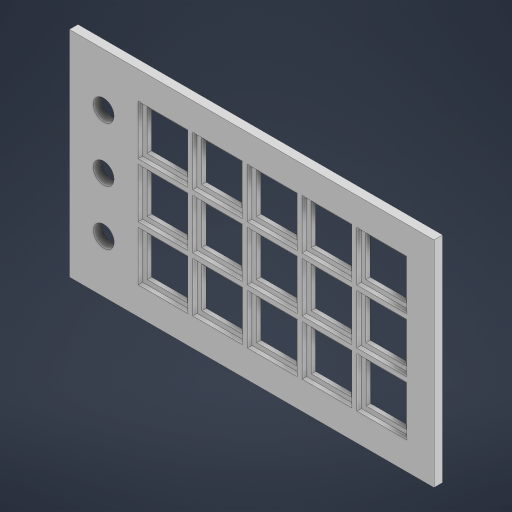
# Autodesk Inventor part: keypadTop
Saved by Autodesk Inventor 2024.3 (Build 283343000, 343)
## iProperties
Created: 2025-12-23
Part Number: keypadTop
Material: Generic
Document SubType Name: Modeling
Designer: zokur
Density: 1 g/cm^3
Appearance: Default
Author: zokur
Autodesk Inventor part; units mm, degrees
ref_plane "YZ Plane" through (0, 0, 0) normal (1, 0, 0) x (0, 1, 0)
ref_plane "XZ Plane" through (0, 0, 0) normal (0, 1, 0) x (-1, 0, 0)
ref_plane "XY Plane" through (0, 0, 0) normal (0, 0, 1) x (1, 0, 0)
sketch "Sketch1" plane through (0, 0, 0) normal (0, 0, 1) x (1, 0, 0)
  line L0 (0, 0) -> (126.85, 0)
  line L1 (126.85, 0) -> (126.85, 74.6)
  line L2 (126.85, 74.6) -> (0, 74.6)
  line L3 (0, 74.6) -> (0, 0)
  line L4 (100, 64.95) -> (117.3, 64.95)
  line L5 (117.3, 64.95) -> (117.3, 47.65)
  line L6 (117.3, 47.65) -> (100, 47.65)
  line L7 (100, 47.65) -> (100, 64.95)
  line L8 (100, 45.95) -> (117.3, 45.95)
  line L9 (117.3, 45.95) -> (117.3, 28.65)
  line L10 (117.3, 28.65) -> (100, 28.65)
  line L11 (100, 28.65) -> (100, 45.95)
  line L12 (100.05, 26.95) -> (117.35, 26.95)
  line L13 (117.35, 26.95) -> (117.35, 9.65)
  line L14 (117.35, 9.65) -> (100.05, 9.65)
  line L15 (100.05, 9.65) -> (100.05, 26.95)
  line L16 (80.95, 65.0676) -> (98.25, 65.0676)
  line L17 (98.25, 65.0676) -> (98.25, 47.7676)
  line L18 (98.25, 47.7676) -> (80.95, 47.7676)
  line L19 (80.95, 47.7676) -> (80.95, 65.0676)
  line L20 (80.95, 46.0676) -> (98.25, 46.0676)
  line L21 (98.25, 46.0676) -> (98.25, 28.7676)
  line L22 (98.25, 28.7676) -> (80.95, 28.7676)
  line L23 (80.95, 28.7676) -> (80.95, 46.0676)
  line L24 (98.3, 27.0676) -> (98.3, 9.7676)
  line L25 (81, 27.0676) -> (98.3, 27.0676)
  line L26 (81, 9.7676) -> (81, 27.0676)
  line L27 (98.3, 9.7676) -> (81, 9.7676)
  line L28 (61.95, 64.95) -> (79.25, 64.95)
  line L29 (79.25, 64.95) -> (79.25, 47.65)
  line L30 (79.25, 47.65) -> (61.95, 47.65)
  line L31 (61.95, 47.65) -> (61.95, 64.95)
  line L32 (61.95, 45.95) -> (79.25, 45.95)
  line L33 (79.25, 45.95) -> (79.25, 28.65)
  line L34 (79.25, 28.65) -> (61.95, 28.65)
  line L35 (61.95, 28.65) -> (61.95, 45.95)
  line L36 (79.3, 26.95) -> (79.3, 9.65)
  line L37 (62, 26.95) -> (79.3, 26.95)
  line L38 (62, 9.65) -> (62, 26.95)
  line L39 (79.3, 9.65) -> (62, 9.65)
  line L40 (60.2, 28.7676) -> (42.9, 28.7676)
  line L41 (42.9, 28.7676) -> (42.9, 46.0676)
  line L42 (60.2, 46.0676) -> (60.2, 28.7676)
  line L43 (42.9, 46.0676) -> (60.2, 46.0676)
  line L44 (60.2, 47.7676) -> (42.9, 47.7676)
  line L45 (60.2, 65.0676) -> (60.2, 47.7676)
  line L46 (42.9, 47.7676) -> (42.9, 65.0676)
  line L47 (42.9, 65.0676) -> (60.2, 65.0676)
  line L48 (42.95, 27.0676) -> (60.25, 27.0676)
  line L49 (42.95, 9.7676) -> (42.95, 27.0676)
  line L50 (60.25, 9.7676) -> (42.95, 9.7676)
  line L51 (60.25, 27.0676) -> (60.25, 9.7676)
  line L52 (41.2, 64.95) -> (41.2, 47.65)
  line L53 (23.9, 64.95) -> (41.2, 64.95)
  line L54 (23.9, 47.65) -> (23.9, 64.95)
  line L55 (41.2, 47.65) -> (23.9, 47.65)
  line L56 (23.9, 45.95) -> (41.2, 45.95)
  line L57 (41.2, 45.95) -> (41.2, 28.65)
  line L58 (23.9, 28.65) -> (23.9, 45.95)
  line L59 (41.2, 28.65) -> (23.9, 28.65)
  line L60 (23.95, 26.95) -> (41.25, 26.95)
  line L61 (41.25, 9.65) -> (23.95, 9.65)
  line L62 (41.25, 26.95) -> (41.25, 9.65)
  line L63 (23.95, 9.65) -> (23.95, 26.95)
  circle A0 centre (11.95, 56.3) radius 3.6
  circle A1 centre (11.95, 37.3) radius 3.6
  circle A2 centre (12, 18.3) radius 3.6
  point P0 (108.65, 45.95)
  point P1 (108.7, 26.95)
  point P2 (89.6, 46.0676)
  point P3 (89.65, 27.0676)
  point P4 (70.6, 45.95)
  point P5 (70.65, 26.95)
  point P6 (51.55, 46.0676)
  point P7 (51.6, 27.0676)
  point P8 (32.55, 45.95)
  point P9 (32.6, 26.95)
  dimension "d0" = 74.6
  dimension "d1" = 126.85
  dimension "d2" = 17.3
  dimension "d3" = 17.3
  dimension "d4" = 9.55
  dimension "d5" = 9.65
  dimension "d6" = 17.3
  dimension "d7" = 17.3
  dimension "d8" = 9.55
  dimension "d9" = 1.7
  dimension "d10" = 17.3
  dimension "d11" = 17.3
  dimension "d12" = 1.7
  dimension "d13" = 9.5
  dimension "d14" = 17.3
  dimension "d15" = 17.3
  dimension "d16" = 17.3
  dimension "d17" = 17.3
  dimension "d18" = 1.7
  dimension "d19" = 17.3
  dimension "d20" = 17.3
  dimension "d21" = 1.7
  dimension "d22" = 1.7
  dimension "d23" = 28.6
  dimension "d24" = 28.6
  dimension "d25" = 0.1176
  dimension "d26" = 17.3
  dimension "d27" = 17.3
  dimension "d28" = 17.3
  dimension "d29" = 17.3
  dimension "d30" = 1.7
  dimension "d31" = 17.3
  dimension "d32" = 17.3
  dimension "d33" = 1.7
  dimension "d34" = 17.3
  dimension "d35" = 17.3
  dimension "d36" = 17.3
  dimension "d37" = 17.3
  dimension "d38" = 1.7
  dimension "d39" = 17.3
  dimension "d40" = 17.3
  dimension "d41" = 1.7
  dimension "d42" = 1.7
  dimension "d43" = 0.1176
  dimension "d44" = 1.7
  dimension "d45" = 1.7
  dimension "d46" = 9.65
  dimension "d47" = 47.6
  dimension "d48" = 66.65
  dimension "d49" = 66.65
  dimension "d50" = 17.3
  dimension "d51" = 17.3
  dimension "d52" = 17.3
  dimension "d53" = 17.3
  dimension "d54" = 1.7
  dimension "d55" = 17.3
  dimension "d56" = 17.3
  dimension "d57" = 1.7
  dimension "d58" = 1.7
  dimension "d59" = 9.65
  dimension "d60" = 85.65
  dimension "d61" = 85.65
  dimension "d62" = 7.2
  dimension "d63" = 11.95
  constraints: 128 end point, 32 parallel, 16 horizontal, 16 perpendicular, 10 midpoint, 3 centre point
  measures "d0" distance of L0.end L1.end
  measures "d1" distance of L1.end L2.end
  measures "d2" distance of L5.end L6.end
  measures "d3" distance of L6.end L4.start
  measures "d4" distance between parallel lines of L1 L5
  measures "d5" distance between parallel lines of L2 L4
  measures "d6" distance of L9.end L10.end
  measures "d7" distance of L10.end L8.start
  measures "d8" distance between parallel lines of L1 L9
  measures "d9" distance from line of point (108.65, 45.95) L6
  measures "d10" distance of L13.end L15.start
  measures "d11" distance of L15.start L12.start
  measures "d12" distance between parallel lines of L12 L10
  measures "d13" distance between parallel lines of L1 L13
  measures "d14" distance of L18.start L18.end
  measures "d15" distance of L18.end L19.end
  measures "d16" distance of L22.start L22.end
  measures "d17" distance of L22.end L23.end
  measures "d18" distance from line of point (89.6, 46.068) L18
  measures "d19" distance of L27.start L26.start
  measures "d20" distance of L26.start L25.start
  measures "d21" distance between parallel lines of L25 L22
  measures "d22" distance between parallel lines of L11 L24
  measures "d23" distance between parallel lines of L17 L1
  measures "d24" distance between parallel lines of L21 L1
  measures "d25" distance between parallel lines of L27 L14
  measures "d26" distance of L30.start L30.end
  measures "d27" distance of L30.end L28.start
  measures "d28" distance of L33.end L35.start
  measures "d29" distance of L35.start L32.start
  measures "d30" distance from line of point (70.6, 45.95) L30
  measures "d31" distance of L36.end L38.start
  measures "d32" distance of L38.start L37.start
  measures "d33" distance between parallel lines of L37 L34
  measures "d34" distance of L45.end L46.start
  measures "d35" distance of L46.start L47.start
  measures "d36" distance of L42.end L41.start
  measures "d37" distance of L41.start L43.start
  measures "d38" distance from line of point (51.55, 46.068) L44
  measures "d39" distance of L50.start L50.end
  measures "d40" distance of L50.end L48.start
  measures "d41" distance between parallel lines of L48 L40
  measures "d42" distance between parallel lines of L35 L51
  measures "d43" distance between parallel lines of L50 L39
  measures "d44" distance between parallel lines of L26 L36
  measures "d45" distance between parallel lines of L23 L33
  measures "d46" distance between parallel lines of L2 L28
  measures "d47" distance between parallel lines of L29 L1
  measures "d48" distance between parallel lines of L45 L1
  measures "d49" distance between parallel lines of L42 L1
  measures "d50" distance of L55.start L55.end
  measures "d51" distance of L55.end L53.start
  measures "d52" distance of L57.end L59.end
  measures "d53" distance of L59.end L56.start
  measures "d54" distance from line of point (32.55, 45.95) L55
  measures "d55" distance of L62.end L61.end
  measures "d56" distance of L61.end L60.start
  measures "d57" distance between parallel lines of L60 L59
  measures "d58" distance between parallel lines of L49 L62
  measures "d59" distance between parallel lines of L0 L61
  measures "d60" distance between parallel lines of L52 L1
  measures "d61" distance between parallel lines of L57 L1
  measures "d62" diameter of A0
  measures "d63" distance from line of L54 A0.centre
extrude "Extrusion1" add sketch "Sketch1" along normal blind 3
sketch "Sketch3" plane through (0, 0, 0) normal (0, 0, -1) x (-1, 0, 0)
  line L0 (-126.85, 0) -> (-126.85, 74.6) projected
  line L1 (0, 0) -> (-126.85, 0) projected
  line L2 (0, 74.6) -> (0, 0) projected
  line L3 (-126.85, 74.6) -> (0, 74.6) projected
  circle A0 centre (-11.95, 56.3) radius 3.6 projected
  circle A1 centre (-11.95, 37.3) radius 3.6 projected
  circle A2 centre (-12, 18.3) radius 3.6 projected
  line L4 (-41.25, 26.95) -> (-41.25, 9.65) projected
  line L5 (-23.95, 26.95) -> (-41.25, 26.95) projected
  line L6 (-23.95, 9.65) -> (-23.95, 26.95) projected
  line L7 (-41.25, 9.65) -> (-23.95, 9.65) projected
  line L8 (-41.2, 47.65) -> (-23.9, 47.65) projected
  line L9 (-41.2, 64.95) -> (-41.2, 47.65) projected
  line L10 (-23.9, 64.95) -> (-41.2, 64.95) projected
  line L11 (-23.9, 47.65) -> (-23.9, 64.95) projected
  line L12 (-41.2, 45.95) -> (-41.2, 28.65) projected
  line L13 (-23.9, 45.95) -> (-41.2, 45.95) projected
  line L14 (-23.9, 28.65) -> (-23.9, 45.95) projected
  line L15 (-41.2, 28.65) -> (-23.9, 28.65) projected
  line L16 (-62, 26.95) -> (-79.3, 26.95) projected
  line L17 (-62, 9.65) -> (-62, 26.95) projected
  line L18 (-79.3, 9.65) -> (-62, 9.65) projected
  line L19 (-79.3, 26.95) -> (-79.3, 9.65) projected
  line L20 (-42.95, 27.0676) -> (-60.25, 27.0676) projected
  line L21 (-42.95, 9.7676) -> (-42.95, 27.0676) projected
  line L22 (-60.25, 9.7676) -> (-42.95, 9.7676) projected
  line L23 (-60.25, 27.0676) -> (-60.25, 9.7676) projected
  line L24 (-61.95, 45.95) -> (-79.25, 45.95) projected
  line L25 (-61.95, 28.65) -> (-61.95, 45.95) projected
  line L26 (-79.25, 28.65) -> (-61.95, 28.65) projected
  line L27 (-79.25, 45.95) -> (-79.25, 28.65) projected
  line L28 (-79.25, 47.65) -> (-61.95, 47.65) projected
  line L29 (-79.25, 64.95) -> (-79.25, 47.65) projected
  line L30 (-61.95, 64.95) -> (-79.25, 64.95) projected
  line L31 (-61.95, 47.65) -> (-61.95, 64.95) projected
  line L32 (-42.9, 46.0676) -> (-60.2, 46.0676) projected
  line L33 (-42.9, 28.7676) -> (-42.9, 46.0676) projected
  line L34 (-60.2, 28.7676) -> (-42.9, 28.7676) projected
  line L35 (-60.2, 46.0676) -> (-60.2, 28.7676) projected
  line L36 (-60.2, 65.0676) -> (-60.2, 47.7676) projected
  line L37 (-42.9, 65.0676) -> (-60.2, 65.0676) projected
  line L38 (-42.9, 47.7676) -> (-42.9, 65.0676) projected
  line L39 (-60.2, 47.7676) -> (-42.9, 47.7676) projected
  line L40 (-81, 27.0676) -> (-98.3, 27.0676) projected
  line L41 (-81, 9.7676) -> (-81, 27.0676) projected
  line L42 (-98.3, 9.7676) -> (-81, 9.7676) projected
  line L43 (-98.3, 27.0676) -> (-98.3, 9.7676) projected
  line L44 (-98.25, 47.7676) -> (-80.95, 47.7676) projected
  line L45 (-98.25, 65.0676) -> (-98.25, 47.7676) projected
  line L46 (-80.95, 65.0676) -> (-98.25, 65.0676) projected
  line L47 (-80.95, 47.7676) -> (-80.95, 65.0676) projected
  line L48 (-98.25, 28.7676) -> (-80.95, 28.7676) projected
  line L49 (-98.25, 46.0676) -> (-98.25, 28.7676) projected
  line L50 (-80.95, 46.0676) -> (-98.25, 46.0676) projected
  line L51 (-80.95, 28.7676) -> (-80.95, 46.0676) projected
  line L52 (-117.35, 26.95) -> (-117.35, 9.65) projected
  line L53 (-100.05, 26.95) -> (-117.35, 26.95) projected
  line L54 (-100.05, 9.65) -> (-100.05, 26.95) projected
  line L55 (-117.35, 9.65) -> (-100.05, 9.65) projected
  line L56 (-100, 45.95) -> (-117.3, 45.95) projected
  line L57 (-100, 28.65) -> (-100, 45.95) projected
  line L58 (-117.3, 28.65) -> (-100, 28.65) projected
  line L59 (-117.3, 45.95) -> (-117.3, 28.65) projected
  line L60 (-100, 64.95) -> (-117.3, 64.95) projected
  line L61 (-100, 47.65) -> (-100, 64.95) projected
  line L62 (-117.3, 47.65) -> (-100, 47.65) projected
  line L63 (-117.3, 64.95) -> (-117.3, 47.65) projected
  line L64 (-115.65, 63.3) -> (-115.65, 49.3) projected
  line L65 (-101.65, 63.3) -> (-115.65, 63.3) projected
  line L66 (-101.65, 49.3) -> (-101.65, 63.3) projected
  line L67 (-115.65, 49.3) -> (-101.65, 49.3) projected
  line L68 (-96.6, 63.4176) -> (-96.6, 49.4176) projected
  line L69 (-82.6, 63.4176) -> (-96.6, 63.4176) projected
  line L70 (-82.6, 49.4176) -> (-82.6, 63.4176) projected
  line L71 (-96.6, 49.4176) -> (-82.6, 49.4176) projected
  line L72 (-77.6, 63.3) -> (-77.6, 49.3) projected
  line L73 (-63.6, 63.3) -> (-77.6, 63.3) projected
  line L74 (-63.6, 49.3) -> (-63.6, 63.3) projected
  line L75 (-77.6, 49.3) -> (-63.6, 49.3) projected
  line L76 (-58.55, 63.4176) -> (-58.55, 49.4176) projected
  line L77 (-44.55, 63.4176) -> (-58.55, 63.4176) projected
  line L78 (-44.55, 49.4176) -> (-44.55, 63.4176) projected
  line L79 (-58.55, 49.4176) -> (-44.55, 49.4176) projected
  line L80 (-39.55, 63.3) -> (-39.55, 49.3) projected
  line L81 (-25.55, 63.3) -> (-39.55, 63.3) projected
  line L82 (-25.55, 49.3) -> (-25.55, 63.3) projected
  line L83 (-39.55, 49.3) -> (-25.55, 49.3) projected
  line L84 (-25.55, 44.3) -> (-39.55, 44.3) projected
  line L85 (-39.55, 44.3) -> (-39.55, 30.3) projected
  line L86 (-39.55, 30.3) -> (-25.55, 30.3) projected
  line L87 (-23.9, 28.65) -> (-23.9, 45.95) projected
  line L88 (-25.55, 30.3) -> (-25.55, 44.3) projected
  line L89 (-58.55, 30.4176) -> (-44.55, 30.4176) projected
  line L90 (-58.55, 44.4176) -> (-58.55, 30.4176) projected
  line L91 (-44.55, 44.4176) -> (-58.55, 44.4176) projected
  line L92 (-44.55, 30.4176) -> (-44.55, 44.4176) projected
  line L93 (-42.9, 28.7676) -> (-42.9, 46.0676) projected
  line L94 (-44.6, 25.4176) -> (-58.6, 25.4176) projected
  line L95 (-58.6, 25.4176) -> (-58.6, 11.4176) projected
  line L96 (-58.6, 11.4176) -> (-44.6, 11.4176) projected
  line L97 (-44.6, 11.4176) -> (-44.6, 25.4176) projected
  line L98 (-39.6, 25.3) -> (-39.6, 11.3) projected
  line L99 (-25.6, 25.3) -> (-39.6, 25.3) projected
  line L100 (-39.6, 11.3) -> (-25.6, 11.3) projected
  line L101 (-25.6, 11.3) -> (-25.6, 25.3) projected
  line L102 (-23.95, 9.65) -> (-23.95, 26.95) projected
  line L103 (-23.95, 26.95) -> (-41.25, 26.95) projected
  line L104 (-23.9, 45.95) -> (-41.2, 45.95) projected
  line L105 (-23.9, 45.95) -> (-41.2, 45.95) projected
  line L106 (-23.9, 45.95) -> (-41.2, 45.95) projected
  line L107 (-23.9, 45.95) -> (-41.2, 45.95) projected
  line L108 (-23.9, 47.65) -> (-23.9, 64.95) projected
  line L109 (-23.9, 64.95) -> (-41.2, 64.95) projected
  line L110 (-62, 26.95) -> (-79.3, 26.95) projected
  line L111 (-62, 26.95) -> (-79.3, 26.95) projected
  line L112 (-62, 26.95) -> (-79.3, 26.95) projected
  line L113 (-62, 26.95) -> (-79.3, 26.95) projected
  line L114 (-79.25, 45.95) -> (-79.25, 28.65) projected
  line L115 (-79.25, 45.95) -> (-79.25, 28.65) projected
  line L116 (-79.25, 45.95) -> (-79.25, 28.65) projected
  line L117 (-79.25, 45.95) -> (-79.25, 28.65) projected
  line L118 (-79.25, 47.65) -> (-61.95, 47.65) projected
  line L119 (-41.2, 47.65) -> (-23.9, 47.65) projected
  line L120 (-23.9, 28.65) -> (-23.9, 45.95) projected
  line L121 (-23.9, 28.65) -> (-23.9, 45.95) projected
  line L122 (-23.9, 28.65) -> (-23.9, 45.95) projected
  line L123 (-23.9, 64.95) -> (-41.2, 64.95) projected
  line L124 (-41.2, 28.65) -> (-23.9, 28.65) projected
  line L125 (-41.2, 28.65) -> (-23.9, 28.65) projected
  line L126 (-23.95, 26.95) -> (-41.25, 26.95) projected
  line L127 (-60.2, 46.0676) -> (-60.2, 28.7676) projected
  line L128 (-41.25, 26.95) -> (-41.25, 9.65) projected
  line L129 (-41.25, 26.95) -> (-41.25, 9.65) projected
  line L130 (-81, 9.7676) -> (-81, 27.0676) projected
  line L131 (-98.3, 9.7676) -> (-81, 9.7676) projected
  line L132 (-81, 27.0676) -> (-98.3, 27.0676) projected
  line L133 (-98.3, 27.0676) -> (-98.3, 9.7676) projected
  line L134 (-61.95, 45.95) -> (-79.25, 45.95) projected
  line L135 (-79.25, 64.95) -> (-79.25, 47.65) projected
  line L136 (-79.3, 9.65) -> (-62, 9.65) projected
  line L137 (-79.3, 9.65) -> (-62, 9.65) projected
  line L138 (-61.95, 28.65) -> (-61.95, 45.95) projected
  line L139 (-61.95, 28.65) -> (-61.95, 45.95) projected
  line L140 (-79.3, 9.65) -> (-62, 9.65) projected
  line L141 (-79.3, 9.65) -> (-62, 9.65) projected
  line L142 (-61.95, 45.95) -> (-79.25, 45.95) projected
  line L143 (-61.95, 45.95) -> (-79.25, 45.95) projected
  line L144 (-79.25, 47.65) -> (-61.95, 47.65) projected
  line L145 (-79.25, 47.65) -> (-61.95, 47.65) projected
  line L146 (-61.95, 64.95) -> (-79.25, 64.95) projected
  line L147 (-61.95, 64.95) -> (-79.25, 64.95) projected
  line L148 (-80.95, 28.7676) -> (-80.95, 46.0676) projected
  line L149 (-80.95, 28.7676) -> (-80.95, 46.0676) projected
  line L150 (-98.25, 46.0676) -> (-98.25, 28.7676) projected
  line L151 (-98.25, 28.7676) -> (-80.95, 28.7676) projected
  line L152 (-98.25, 28.7676) -> (-80.95, 28.7676) projected
  line L153 (-98.25, 46.0676) -> (-98.25, 28.7676) projected
  line L154 (-80.95, 46.0676) -> (-98.25, 46.0676) projected
  line L155 (-80.95, 46.0676) -> (-98.25, 46.0676) projected
  line L156 (-98.25, 65.0676) -> (-98.25, 47.7676) projected
  line L157 (-61.95, 47.65) -> (-61.95, 64.95) projected
  line L158 (-61.95, 47.65) -> (-61.95, 64.95) projected
  line L159 (-100, 28.65) -> (-100, 45.95) projected
  line L160 (-80.95, 65.0676) -> (-98.25, 65.0676) projected
  line L161 (-117.35, 26.95) -> (-117.35, 9.65) projected
  line L162 (-117.35, 26.95) -> (-117.35, 9.65) projected
  line L163 (-100.05, 9.65) -> (-100.05, 26.95) projected
  line L164 (-100.05, 9.65) -> (-100.05, 26.95) projected
  line L165 (-100.05, 26.95) -> (-117.35, 26.95) projected
  line L166 (-117.35, 9.65) -> (-100.05, 9.65) projected
  line L167 (-117.35, 9.65) -> (-100.05, 9.65) projected
  line L168 (-100, 28.65) -> (-100, 45.95) projected
  line L169 (-117.3, 28.65) -> (-100, 28.65) projected
  line L170 (-117.3, 28.65) -> (-100, 28.65) projected
  line L171 (-79.3, 26.95) -> (-79.3, 9.65) projected
  line L172 (-79.3, 26.95) -> (-79.3, 9.65) projected
  line L173 (-100, 45.95) -> (-117.3, 45.95) projected
  line L174 (-100, 45.95) -> (-117.3, 45.95) projected
  line L175 (-117.3, 45.95) -> (-117.3, 28.65) projected
  line L176 (-117.3, 45.95) -> (-117.3, 28.65) projected
  line L177 (-100.05, 26.95) -> (-117.35, 26.95) projected
  line L178 (-79.3, 26.95) -> (-79.3, 9.65) projected
  line L179 (-79.3, 26.95) -> (-79.3, 9.65) projected
  line L180 (-79.25, 64.95) -> (-79.25, 47.65) projected
  line L181 (-79.25, 64.95) -> (-79.25, 47.65) projected
  line L182 (-80.95, 47.7676) -> (-80.95, 65.0676) projected
  line L183 (-80.95, 47.7676) -> (-80.95, 65.0676) projected
  line L184 (-80.95, 28.7676) -> (-80.95, 46.0676) projected
  line L185 (-80.95, 28.7676) -> (-80.95, 46.0676) projected
  line L186 (-80.95, 65.0676) -> (-98.25, 65.0676) projected
  line L187 (-80.95, 65.0676) -> (-98.25, 65.0676) projected
  line L188 (-98.25, 65.0676) -> (-98.25, 47.7676) projected
  line L189 (-98.25, 65.0676) -> (-98.25, 47.7676) projected
  line L190 (-80.95, 46.0676) -> (-98.25, 46.0676) projected
  line L191 (-80.95, 46.0676) -> (-98.25, 46.0676) projected
  line L192 (-98.25, 47.7676) -> (-80.95, 47.7676) projected
  line L193 (-98.25, 47.7676) -> (-80.95, 47.7676) projected
  line L194 (-100, 47.65) -> (-100, 64.95) projected
  line L195 (-100, 47.65) -> (-100, 64.95) projected
  line L196 (-100, 64.95) -> (-117.3, 64.95) projected
  line L197 (-100, 64.95) -> (-117.3, 64.95) projected
  line L198 (-117.3, 64.95) -> (-117.3, 47.65) projected
  line L199 (-117.3, 64.95) -> (-117.3, 47.65) projected
  line L200 (-98.25, 28.7676) -> (-80.95, 28.7676) projected
  line L201 (-98.25, 28.7676) -> (-80.95, 28.7676) projected
  line L202 (-98.25, 46.0676) -> (-98.25, 28.7676) projected
  line L203 (-98.25, 46.0676) -> (-98.25, 28.7676) projected
  line L204 (-81, 9.7676) -> (-81, 27.0676) projected
  line L205 (-81, 9.7676) -> (-81, 27.0676) projected
  line L206 (-81, 27.0676) -> (-98.3, 27.0676) projected
  line L207 (-81, 27.0676) -> (-98.3, 27.0676) projected
  line L208 (-100, 28.65) -> (-100, 45.95) projected
  line L209 (-100, 28.65) -> (-100, 45.95) projected
  line L210 (-98.3, 9.7676) -> (-81, 9.7676) projected
  line L211 (-98.3, 9.7676) -> (-81, 9.7676) projected
  line L212 (-117.3, 47.65) -> (-100, 47.65) projected
  line L213 (-117.3, 47.65) -> (-100, 47.65) projected
  line L214 (-100, 45.95) -> (-117.3, 45.95) projected
  line L215 (-100, 45.95) -> (-117.3, 45.95) projected
  line L216 (-117.3, 45.95) -> (-117.3, 28.65) projected
  line L217 (-117.3, 45.95) -> (-117.3, 28.65) projected
  line L218 (-98.3, 27.0676) -> (-98.3, 9.7676) projected
  line L219 (-98.3, 27.0676) -> (-98.3, 9.7676) projected
  line L220 (-117.3, 28.65) -> (-100, 28.65) projected
  line L221 (-117.3, 28.65) -> (-100, 28.65) projected
  line L222 (-100.05, 26.95) -> (-117.35, 26.95) projected
  line L223 (-100.05, 26.95) -> (-117.35, 26.95) projected
  line L224 (-117.35, 26.95) -> (-117.35, 9.65) projected
  line L225 (-117.35, 26.95) -> (-117.35, 9.65) projected
  line L226 (-117.35, 9.65) -> (-100.05, 9.65) projected
  line L227 (-117.35, 9.65) -> (-100.05, 9.65) projected
  line L228 (-100.05, 9.65) -> (-100.05, 26.95) projected
  line L229 (-100.05, 9.65) -> (-100.05, 26.95) projected
  line L230 (-100, 47.65) -> (-100, 64.95) projected
  line L231 (-117.3, 64.95) -> (-117.3, 47.65) projected
  line L232 (-117.3, 64.95) -> (-117.3, 47.65) projected
  line L233 (-100, 47.65) -> (-100, 64.95) projected
  line L234 (-117.3, 47.65) -> (-100, 47.65) projected
  line L235 (-100, 64.95) -> (-117.3, 64.95) projected
  line L236 (-100, 64.95) -> (-117.3, 64.95) projected
  line L237 (-98.25, 65.0676) -> (-98.25, 47.7676) projected
  line L238 (-98.25, 47.7676) -> (-80.95, 47.7676) projected
  line L239 (-98.25, 47.7676) -> (-80.95, 47.7676) projected
  line L240 (-61.95, 47.65) -> (-61.95, 64.95) projected
  line L241 (-60.2, 47.7676) -> (-42.9, 47.7676) projected
  line L242 (-60.2, 28.7676) -> (-42.9, 28.7676) projected
  line L243 (-60.2, 28.7676) -> (-42.9, 28.7676) projected
  line L244 (-41.2, 64.95) -> (-41.2, 47.65) projected
  line L245 (-41.2, 64.95) -> (-41.2, 47.65) projected
  line L246 (-60.2, 47.7676) -> (-42.9, 47.7676) projected
  line L247 (-60.2, 47.7676) -> (-42.9, 47.7676) projected
  line L248 (-60.2, 47.7676) -> (-42.9, 47.7676) projected
  line L249 (-42.9, 65.0676) -> (-60.2, 65.0676) projected
  line L250 (-41.2, 45.95) -> (-41.2, 28.65) projected
  line L251 (-41.2, 45.95) -> (-41.2, 28.65) projected
  line L252 (-41.2, 45.95) -> (-41.2, 28.65) projected
  line L253 (-41.2, 45.95) -> (-41.2, 28.65) projected
  line L254 (-23.9, 47.65) -> (-23.9, 64.95) projected
  line L255 (-61.95, 45.95) -> (-79.25, 45.95) projected
  line L256 (-60.25, 27.0676) -> (-60.25, 9.7676) projected
  line L257 (-60.25, 27.0676) -> (-60.25, 9.7676) projected
  line L258 (-60.25, 27.0676) -> (-60.25, 9.7676) projected
  line L259 (-60.25, 27.0676) -> (-60.25, 9.7676) projected
  line L260 (-42.95, 9.7676) -> (-42.95, 27.0676) projected
  line L261 (-60.25, 9.7676) -> (-42.95, 9.7676) projected
  line L262 (-60.25, 9.7676) -> (-42.95, 9.7676) projected
  line L263 (-42.95, 27.0676) -> (-60.25, 27.0676) projected
  line L264 (-42.95, 27.0676) -> (-60.25, 27.0676) projected
  line L265 (-42.95, 27.0676) -> (-60.25, 27.0676) projected
  line L266 (-42.95, 27.0676) -> (-60.25, 27.0676) projected
  line L267 (-60.2, 46.0676) -> (-60.2, 28.7676) projected
  line L268 (-61.95, 28.65) -> (-61.95, 45.95) projected
  line L269 (-62, 9.65) -> (-62, 26.95) projected
  line L270 (-61.95, 28.65) -> (-61.95, 45.95) projected
  line L271 (-62, 9.65) -> (-62, 26.95) projected
  line L272 (-62, 9.65) -> (-62, 26.95) projected
  line L273 (-62, 9.65) -> (-62, 26.95) projected
  line L274 (-41.25, 9.65) -> (-23.95, 9.65) projected
  line L275 (-41.25, 9.65) -> (-23.95, 9.65) projected
  line L276 (-23.95, 9.65) -> (-23.95, 26.95) projected
  line L277 (-41.2, 47.65) -> (-23.9, 47.65) projected
  line L278 (-42.9, 46.0676) -> (-60.2, 46.0676) projected
  line L279 (-42.9, 46.0676) -> (-60.2, 46.0676) projected
  line L280 (-42.9, 46.0676) -> (-60.2, 46.0676) projected
  line L281 (-42.9, 46.0676) -> (-60.2, 46.0676) projected
  line L282 (-80.95, 65.0676) -> (-98.25, 65.0676) projected
  line L283 (-81, 27.0676) -> (-98.3, 27.0676) projected
  line L284 (-98.3, 9.7676) -> (-81, 9.7676) projected
  line L285 (-98.3, 27.0676) -> (-98.3, 9.7676) projected
  line L286 (-81, 9.7676) -> (-81, 27.0676) projected
  line L287 (-79.25, 28.65) -> (-61.95, 28.65) projected
  line L288 (-79.25, 28.65) -> (-61.95, 28.65) projected
  line L289 (-79.25, 28.65) -> (-61.95, 28.65) projected
  line L290 (-79.25, 28.65) -> (-61.95, 28.65) projected
  line L291 (-79.25, 47.65) -> (-61.95, 47.65) projected
  line L292 (-79.25, 64.95) -> (-79.25, 47.65) projected
  line L293 (-61.95, 47.65) -> (-61.95, 64.95) projected
  line L294 (-61.95, 64.95) -> (-79.25, 64.95) projected
  line L295 (-61.95, 64.95) -> (-79.25, 64.95) projected
  line L296 (-60.2, 65.0676) -> (-60.2, 47.7676) projected
  line L297 (-60.2, 65.0676) -> (-60.2, 47.7676) projected
  line L298 (-60.2, 65.0676) -> (-60.2, 47.7676) projected
  line L299 (-80.95, 47.7676) -> (-80.95, 65.0676) projected
  line L300 (-80.95, 47.7676) -> (-80.95, 65.0676) projected
  line L301 (-60.2, 65.0676) -> (-60.2, 47.7676) projected
  line L302 (-42.9, 65.0676) -> (-60.2, 65.0676) projected
  line L303 (-42.9, 28.7676) -> (-42.9, 46.0676) projected
  line L304 (-42.95, 9.7676) -> (-42.95, 27.0676) projected
  line L305 (-60.2, 46.0676) -> (-60.2, 28.7676) projected
  line L306 (-60.2, 46.0676) -> (-60.2, 28.7676) projected
  line L307 (-60.25, 9.7676) -> (-42.95, 9.7676) projected
  line L308 (-60.25, 9.7676) -> (-42.95, 9.7676) projected
  line L309 (-42.9, 65.0676) -> (-60.2, 65.0676) projected
  line L310 (-42.9, 65.0676) -> (-60.2, 65.0676) projected
  line L311 (-42.9, 47.7676) -> (-42.9, 65.0676) projected
  line L312 (-42.9, 47.7676) -> (-42.9, 65.0676) projected
  line L313 (-42.9, 47.7676) -> (-42.9, 65.0676) projected
  line L314 (-42.9, 47.7676) -> (-42.9, 65.0676) projected
  line L315 (-42.9, 28.7676) -> (-42.9, 46.0676) projected
  line L316 (-42.9, 28.7676) -> (-42.9, 46.0676) projected
  line L317 (-41.2, 64.95) -> (-41.2, 47.65) projected
  line L318 (-41.2, 64.95) -> (-41.2, 47.65) projected
  line L319 (-23.9, 64.95) -> (-41.2, 64.95) projected
  line L320 (-23.9, 64.95) -> (-41.2, 64.95) projected
  line L321 (-41.2, 47.65) -> (-23.9, 47.65) projected
  line L322 (-41.2, 47.65) -> (-23.9, 47.65) projected
  line L323 (-23.9, 47.65) -> (-23.9, 64.95) projected
  line L324 (-23.9, 47.65) -> (-23.9, 64.95) projected
  line L325 (-41.25, 26.95) -> (-41.25, 9.65) projected
  line L326 (-41.25, 26.95) -> (-41.25, 9.65) projected
  line L327 (-41.25, 9.65) -> (-23.95, 9.65) projected
  line L328 (-41.25, 9.65) -> (-23.95, 9.65) projected
  line L329 (-42.95, 9.7676) -> (-42.95, 27.0676) projected
  line L330 (-42.95, 9.7676) -> (-42.95, 27.0676) projected
  line L331 (-23.95, 26.95) -> (-41.25, 26.95) projected
  line L332 (-23.95, 26.95) -> (-41.25, 26.95) projected
  line L333 (-23.95, 9.65) -> (-23.95, 26.95) projected
  line L334 (-23.95, 9.65) -> (-23.95, 26.95) projected
  line L335 (-41.2, 28.65) -> (-23.9, 28.65) projected
  line L336 (-41.2, 28.65) -> (-23.9, 28.65) projected
  line L337 (-60.2, 28.7676) -> (-42.9, 28.7676) projected
  line L338 (-60.2, 28.7676) -> (-42.9, 28.7676) projected
  line L339 (-117.3, 47.65) -> (-100, 47.65) projected
  line L340 (-117.35, 26.95) -> (-117.35, 9.65) projected
  line L341 (-117.35, 9.65) -> (-100.05, 9.65) projected
  line L342 (-100.05, 9.65) -> (-100.05, 26.95) projected
  line L343 (-96.65, 25.4176) -> (-96.65, 11.4176) projected
  line L344 (-101.7, 25.3) -> (-115.7, 25.3) projected
  line L345 (-101.7, 11.3) -> (-101.7, 25.3) projected
  line L346 (-115.7, 11.3) -> (-101.7, 11.3) projected
  line L347 (-115.7, 25.3) -> (-115.7, 11.3) projected
  line L348 (-96.6, 44.4176) -> (-96.6, 30.4176) projected
  line L349 (-101.65, 30.3) -> (-101.65, 44.3) projected
  line L350 (-115.65, 30.3) -> (-101.65, 30.3) projected
  line L351 (-100, 28.65) -> (-100, 45.95) projected
  line L352 (-100.05, 26.95) -> (-117.35, 26.95) projected
  line L353 (-117.3, 28.65) -> (-100, 28.65) projected
  line L354 (-101.65, 44.3) -> (-115.65, 44.3) projected
  line L355 (-115.65, 44.3) -> (-115.65, 30.3) projected
  line L356 (-117.3, 45.95) -> (-117.3, 28.65) projected
  line L357 (-100, 45.95) -> (-117.3, 45.95) projected
  line L358 (-98.25, 46.0676) -> (-98.25, 28.7676) projected
  line L359 (-81, 27.0676) -> (-98.3, 27.0676) projected
  line L360 (-98.3, 27.0676) -> (-98.3, 9.7676) projected
  line L361 (-98.3, 9.7676) -> (-81, 9.7676) projected
  line L362 (-81, 9.7676) -> (-81, 27.0676) projected
  line L363 (-98.25, 28.7676) -> (-80.95, 28.7676) projected
  line L364 (-80.95, 46.0676) -> (-98.25, 46.0676) projected
  line L365 (-80.95, 28.7676) -> (-80.95, 46.0676) projected
  line L366 (-82.6, 44.4176) -> (-96.6, 44.4176) projected
  line L367 (-82.6, 30.4176) -> (-82.6, 44.4176) projected
  line L368 (-96.6, 30.4176) -> (-82.6, 30.4176) projected
  line L369 (-82.65, 25.4176) -> (-96.65, 25.4176) projected
  line L370 (-96.65, 11.4176) -> (-82.65, 11.4176) projected
  line L371 (-82.65, 11.4176) -> (-82.65, 25.4176) projected
  line L372 (-98.25, 47.7676) -> (-80.95, 47.7676) projected
  line L373 (-80.95, 47.7676) -> (-80.95, 65.0676) projected
  line L374 (-80.95, 65.0676) -> (-98.25, 65.0676) projected
  line L375 (-98.25, 65.0676) -> (-98.25, 47.7676) projected
  line L376 (-100, 64.95) -> (-117.3, 64.95) projected
  line L377 (-117.3, 64.95) -> (-117.3, 47.65) projected
  line L378 (-117.3, 47.65) -> (-100, 47.65) projected
  line L379 (-100, 47.65) -> (-100, 64.95) projected
  line L380 (-77.65, 25.3) -> (-77.65, 11.3) projected
  line L381 (-79.3, 26.95) -> (-79.3, 9.65) projected
  line L382 (-62, 9.65) -> (-62, 26.95) projected
  line L383 (-63.65, 11.3) -> (-63.65, 25.3) projected
  line L384 (-77.65, 11.3) -> (-63.65, 11.3) projected
  line L385 (-79.3, 9.65) -> (-62, 9.65) projected
  line L386 (-62, 26.95) -> (-79.3, 26.95) projected
  line L387 (-61.95, 45.95) -> (-79.25, 45.95) projected
  line L388 (-79.25, 45.95) -> (-79.25, 28.65) projected
  line L389 (-79.25, 28.65) -> (-61.95, 28.65) projected
  line L390 (-61.95, 28.65) -> (-61.95, 45.95) projected
  line L391 (-63.65, 25.3) -> (-77.65, 25.3) projected
  line L392 (-60.2, 46.0676) -> (-60.2, 28.7676) projected
  line L393 (-63.6, 30.3) -> (-63.6, 44.3) projected
  line L394 (-77.6, 30.3) -> (-63.6, 30.3) projected
  line L395 (-77.6, 44.3) -> (-77.6, 30.3) projected
  line L396 (-63.6, 44.3) -> (-77.6, 44.3) projected
  line L397 (-60.25, 27.0676) -> (-60.25, 9.7676) projected
  line L398 (-60.25, 9.7676) -> (-42.95, 9.7676) projected
  line L399 (-42.95, 9.7676) -> (-42.95, 27.0676) projected
  line L400 (-42.95, 27.0676) -> (-60.25, 27.0676) projected
  line L401 (-60.2, 28.7676) -> (-42.9, 28.7676) projected
  line L402 (-41.25, 26.95) -> (-41.25, 9.65) projected
  line L403 (-41.25, 9.65) -> (-23.95, 9.65) projected
  line L404 (-23.95, 9.65) -> (-23.95, 26.95) projected
  line L405 (-23.95, 26.95) -> (-41.25, 26.95) projected
  line L406 (-41.2, 47.65) -> (-23.9, 47.65) projected
  line L407 (-23.9, 47.65) -> (-23.9, 64.95) projected
  line L408 (-23.9, 64.95) -> (-41.2, 64.95) projected
  line L409 (-41.2, 64.95) -> (-41.2, 47.65) projected
  line L410 (-41.2, 45.95) -> (-41.2, 28.65) projected
  line L411 (-41.2, 28.65) -> (-23.9, 28.65) projected
  line L412 (-23.9, 28.65) -> (-23.9, 45.95) projected
  line L413 (-23.9, 45.95) -> (-41.2, 45.95) projected
  line L414 (-42.9, 28.7676) -> (-42.9, 46.0676) projected
  line L415 (-79.25, 47.65) -> (-61.95, 47.65) projected
  line L416 (-61.95, 47.65) -> (-61.95, 64.95) projected
  line L417 (-61.95, 64.95) -> (-79.25, 64.95) projected
  line L418 (-79.25, 64.95) -> (-79.25, 47.65) projected
  line L419 (-42.9, 46.0676) -> (-60.2, 46.0676) projected
  line L420 (-60.2, 65.0676) -> (-60.2, 47.7676) projected
  line L421 (-60.2, 47.7676) -> (-42.9, 47.7676) projected
  line L422 (-42.9, 47.7676) -> (-42.9, 65.0676) projected
  line L423 (-42.9, 65.0676) -> (-60.2, 65.0676) projected
  point P0 (-98.25, 37.4176)
  point P1 (-108.7, 26.95)
  point P2 (-108.65, 44.3)
  point P3 (-89.65, 27.0676)
  point P4 (-96.6, 56.4176)
  point P5 (-58.6, 18.4176)
  point P6 (-32.6, 26.95)
  point P7 (-32.55, 49.3)
  constraints: 89 other
extrude "Extrusion2" add sketch "Sketch3" against normal blind 1.5 contours L5 L6 L7 L4 | L9 L10 L11 L8 | L13 L14 L15 L12 | L17 L18 L19 L16 | L21 L22 L23 L20 | L25 L26 L27 L24 | L29 L30 L31 L28 | L33 L34 L35 L32 | L37 L38 L39 L36 | L41 L42 L43 L40 | L45 L46 L47 L44 | L49 L50 L51 L48 | L53 L54 L55 L52 | L57 L58 L59 L56 | L61 L62 L63 L60
body "Solid1"
